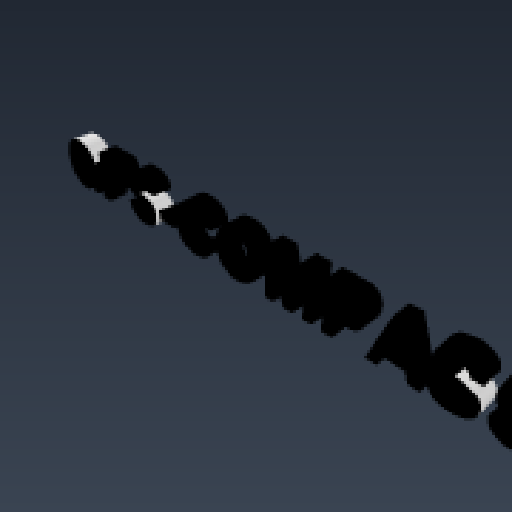
# Autodesk Inventor part: GPS-Compass_name
Saved by Autodesk Inventor 2026.2 (Build 302298000, 298)
## iProperties
Created: 2025-11-27
Part Number: GPS-Compass_name
Material: Generic
Document SubType Name: Modeling
Designer: MenMe
Density: 1 g/cm^3
Appearance: Default
Author: MenMe
Autodesk Inventor part; units mm, degrees
ref_plane "YZ Plane" through (0, 0, 0) normal (1, 0, 0) x (0, 1, 0)
ref_plane "XZ Plane" through (0, 0, 0) normal (0, 1, 0) x (-1, 0, 0)
ref_plane "XY Plane" through (0, 0, 0) normal (0, 0, 1) x (1, 0, 0)
sketch "Sketch2" plane through (0, 0, 0) normal (0, 0, 1) x (1, 0, 0)
  line L0 (0, 0) -> (50, 0) construction
  line L1 (50, 0) -> (50, -7) construction
  line L2 (50, -7) -> (0, -7) construction
  line L3 (0, -7) -> (0, 0) construction
  spline S0 degree 2 poles (4.1164, -4.544) (3.8396, -4.9226) (3.127, -5.2769) (2.6507, -5.2769) knots 0 0 0 1 2 2 2
  spline S1 degree 2 poles (2.6507, -5.2769) (1.6002, -5.2769) (0.2972, -3.8192) (0.2972, -2.6344) knots 0 0 0 1 2 2 2
  spline S2 degree 2 poles (0.2972, -2.6344) (0.2972, -1.4414) (1.5961, -0.0081) (2.6751, -0.0081) knots 0 0 0 1 2 2 2
  spline S3 degree 2 poles (2.6751, -0.0081) (3.6156, -0.0081) (4.8046, -0.908) (4.9186, -1.6938) knots 0 0 0 1 2 2 2
  line L4 (4.9186, -1.6938) -> (3.8681, -1.6938)
  spline S4 degree 2 poles (3.8681, -1.6938) (3.7744, -1.307) (3.184, -0.8998) (2.7117, -0.8998) knots 0 0 0 1 2 2 2
  spline S5 degree 2 poles (2.7117, -0.8998) (2.0847, -0.8998) (1.3681, -1.82) (1.3681, -2.6303) knots 0 0 0 1 2 2 2
  spline S6 degree 2 poles (1.3681, -2.6303) (1.3681, -3.4446) (2.1173, -4.3648) (2.7687, -4.3648) knots 0 0 0 1 2 2 2
  spline S7 degree 2 poles (2.7687, -4.3648) (3.2573, -4.3648) (3.9169, -3.7866) (3.9943, -3.2858) knots 0 0 0 1 2 2 2
  line L5 (3.9943, -3.2858) -> (2.8583, -3.2858)
  line L6 (2.8583, -3.2858) -> (2.8583, -2.4308)
  line L7 (2.8583, -2.4308) -> (4.9308, -2.4308)
  line L8 (4.9308, -2.4308) -> (4.9308, -5.1384)
  line L9 (4.9308, -5.1384) -> (4.2427, -5.1384)
  line L10 (4.2427, -5.1384) -> (4.1164, -4.544)
  line L11 (6.9503, -3.3591) -> (6.9503, -5.1384)
  line L12 (6.9503, -5.1384) -> (5.9202, -5.1384)
  line L13 (5.9202, -5.1384) -> (5.9202, -0.1384)
  line L14 (5.9202, -0.1384) -> (8.1433, -0.1384)
  spline S8 degree 2 poles (8.1433, -0.1384) (8.9332, -0.1384) (9.7435, -0.9568) (9.7435, -1.7467) knots 0 0 0 1 2 2 2
  spline S9 degree 2 poles (9.7435, -1.7467) (9.7435, -2.5204) (8.9495, -3.3591) (8.2125, -3.3591) knots 0 0 0 1 2 2 2
  line L15 (8.2125, -3.3591) -> (6.9503, -3.3591)
  line L16 (6.9585, -2.4511) -> (7.952, -2.4511)
  spline S10 degree 2 poles (7.952, -2.4511) (8.355, -2.4511) (8.7215, -2.1091) (8.7215, -1.7305) knots 0 0 0 1 2 2 2
  spline S11 degree 2 poles (8.7215, -1.7305) (8.7215, -1.3762) (8.3632, -1.0098) (8.0049, -1.0098) knots 0 0 0 1 2 2 2
  line L17 (8.0049, -1.0098) -> (6.9585, -1.0098)
  line L18 (6.9585, -1.0098) -> (6.9585, -2.4511)
  line L19 (10.3298, -3.5912) -> (11.3436, -3.5912)
  spline S12 degree 2 poles (11.3436, -3.5912) (11.4007, -4.0024) (11.9585, -4.4015) (12.4837, -4.4015) knots 0 0 0 1 2 2 2
  spline S13 degree 2 poles (12.4837, -4.4015) (12.9316, -4.4015) (13.3876, -4.0839) (13.3876, -3.7704) knots 0 0 0 1 2 2 2
  spline S14 degree 2 poles (13.3876, -3.7704) (13.3876, -3.3143) (12.0806, -3.013) knots 0 0 0 1 1 1
  spline S15 degree 2 poles (12.0806, -3.013) (12.0603, -3.013) (12.048, -3.009) knots 0 0 0 1 1 1
  spline S16 degree 2 poles (12.048, -3.009) (12.0155, -3.0008) (11.9422, -2.9845) knots 0 0 0 1 1 1
  spline S17 degree 2 poles (11.9422, -2.9845) (11.2459, -2.8298) (10.9446, -2.6425) knots 0 0 0 1 1 1
  spline S18 degree 2 poles (10.9446, -2.6425) (10.68, -2.4715) (10.4031, -1.8974) (10.4031, -1.5065) knots 0 0 0 1 2 2 2
  spline S19 degree 2 poles (10.4031, -1.5065) (10.4031, -0.7777) (11.3925, 0) (12.3331, 0) knots 0 0 0 1 2 2 2
  spline S20 degree 2 poles (12.3331, 0) (13.2085, 0) (14.1938, -0.8306) (14.2223, -1.5839) knots 0 0 0 1 2 2 2
  line L20 (14.2223, -1.5839) -> (13.2329, -1.5839)
  spline S21 degree 2 poles (13.2329, -1.5839) (13.2044, -1.2215) (12.7036, -0.8388) (12.2394, -0.8388) knots 0 0 0 1 2 2 2
  spline S22 degree 2 poles (12.2394, -0.8388) (11.8363, -0.8388) (11.3966, -1.1564) (11.3966, -1.4454) knots 0 0 0 1 2 2 2
  spline S23 degree 2 poles (11.3966, -1.4454) (11.3966, -1.8445) (12.2476, -2.0399) knots 0 0 0 1 1 1
  spline S24 degree 2 poles (12.2476, -2.0399) (12.4796, -2.0969) (12.6099, -2.1254) knots 0 0 0 1 1 1
  spline S25 degree 2 poles (12.6099, -2.1254) (13.1555, -2.2638) (13.6156, -2.4226) (13.7866, -2.5163) knots 0 0 0 1 2 2 2
  spline S26 degree 2 poles (13.7866, -2.5163) (14.092, -2.6873) (14.3974, -3.2451) (14.3974, -3.636) knots 0 0 0 1 2 2 2
  spline S27 degree 2 poles (14.3974, -3.636) (14.3974, -4.4178) (13.3469, -5.2769) (12.386, -5.2769) knots 0 0 0 1 2 2 2
  spline S28 degree 2 poles (12.386, -5.2769) (11.4454, -5.2769) (10.3705, -4.4015) (10.3298, -3.5912) knots 0 0 0 1 2 2 2
  line L21 (14.8941, -3.7541) -> (14.8941, -2.8217)
  line L22 (14.8941, -2.8217) -> (16.8037, -2.8217)
  line L23 (16.8037, -2.8217) -> (16.8037, -3.7541)
  line L24 (16.8037, -3.7541) -> (14.8941, -3.7541)
  spline S29 degree 2 poles (21.8811, -3.4202) (21.8241, -4.2712) (20.623, -5.2769) (19.6621, -5.2769) knots 0 0 0 1 2 2 2
  spline S30 degree 2 poles (19.6621, -5.2769) (18.5505, -5.2769) (17.3168, -3.8925) (17.3168, -2.6425) knots 0 0 0 1 2 2 2
  spline S31 degree 2 poles (17.3168, -2.6425) (17.3168, -1.364) (18.5749, -0.0081) (19.7516, -0.0081) knots 0 0 0 1 2 2 2
  spline S32 degree 2 poles (19.7516, -0.0081) (20.7085, -0.0081) (21.82, -0.9446) (21.873, -1.7956) knots 0 0 0 1 2 2 2
  line L25 (21.873, -1.7956) -> (20.8591, -1.7956)
  spline S33 degree 2 poles (20.8591, -1.7956) (20.794, -1.3681) (20.2321, -0.9243) (19.7516, -0.9243) knots 0 0 0 1 2 2 2
  spline S34 degree 2 poles (19.7516, -0.9243) (19.0717, -0.9243) (18.3673, -1.7997) (18.3673, -2.6425) knots 0 0 0 1 2 2 2
  spline S35 degree 2 poles (18.3673, -2.6425) (18.3673, -3.4568) (19.0717, -4.3445) (19.7191, -4.3445) knots 0 0 0 1 2 2 2
  spline S36 degree 2 poles (19.7191, -4.3445) (20.1873, -4.3445) (20.7818, -3.8681) (20.8713, -3.4202) knots 0 0 0 1 2 2 2
  line L26 (20.8713, -3.4202) -> (21.8811, -3.4202)
  spline S37 degree 2 poles (22.4837, -2.6425) (22.4837, -1.4292) (23.8029, -0.0081) (24.9267, -0.0081) knots 0 0 0 1 2 2 2
  spline S38 degree 2 poles (24.9267, -0.0081) (26.0464, -0.0081) (27.3738, -1.4332) (27.3738, -2.6425) knots 0 0 0 1 2 2 2
  spline S39 degree 2 poles (27.3738, -2.6425) (27.3738, -3.8518) (26.0464, -5.2769) (24.9267, -5.2769) knots 0 0 0 1 2 2 2
  spline S40 degree 2 poles (24.9267, -5.2769) (23.8029, -5.2769) (22.4837, -3.8518) (22.4837, -2.6425) knots 0 0 0 1 2 2 2
  spline S41 degree 2 poles (23.5342, -2.6425) (23.5342, -3.4691) (24.2671, -4.3811) (24.9267, -4.3811) knots 0 0 0 1 2 2 2
  spline S42 degree 2 poles (24.9267, -4.3811) (25.5904, -4.3811) (26.3314, -3.4691) (26.3314, -2.6425) knots 0 0 0 1 2 2 2
  spline S43 degree 2 poles (26.3314, -2.6425) (26.3314, -1.816) (25.5904, -0.9039) (24.9267, -0.9039) knots 0 0 0 1 2 2 2
  spline S44 degree 2 poles (24.9267, -0.9039) (24.2671, -0.9039) (23.5342, -1.8119) (23.5342, -2.6425) knots 0 0 0 1 2 2 2
  line L27 (28.1922, -5.1384) -> (28.1922, -0.1384)
  line L28 (28.1922, -0.1384) -> (29.715, -0.1384)
  line L29 (29.715, -0.1384) -> (30.7125, -3.9454)
  line L30 (30.7125, -3.9454) -> (31.6938, -0.1384)
  line L31 (31.6938, -0.1384) -> (33.2207, -0.1384)
  line L32 (33.2207, -0.1384) -> (33.2207, -5.1384)
  line L33 (33.2207, -5.1384) -> (32.2557, -5.1384)
  line L34 (32.2557, -5.1384) -> (32.2557, -1.1075)
  line L35 (32.2557, -1.1075) -> (31.2419, -5.1384)
  line L36 (31.2419, -5.1384) -> (30.1873, -5.1384)
  line L37 (30.1873, -5.1384) -> (29.1572, -1.1075)
  line L38 (29.1572, -1.1075) -> (29.1572, -5.1384)
  line L39 (29.1572, -5.1384) -> (28.1922, -5.1384)
  line L40 (35.2891, -3.3591) -> (35.2891, -5.1384)
  line L41 (35.2891, -5.1384) -> (34.259, -5.1384)
  line L42 (34.259, -5.1384) -> (34.259, -0.1384)
  line L43 (34.259, -0.1384) -> (36.4821, -0.1384)
  spline S45 degree 2 poles (36.4821, -0.1384) (37.272, -0.1384) (38.0822, -0.9568) (38.0822, -1.7467) knots 0 0 0 1 2 2 2
  spline S46 degree 2 poles (38.0822, -1.7467) (38.0822, -2.5204) (37.2883, -3.3591) (36.5513, -3.3591) knots 0 0 0 1 2 2 2
  line L44 (36.5513, -3.3591) -> (35.2891, -3.3591)
  line L45 (35.2972, -2.4511) -> (36.2907, -2.4511)
  spline S47 degree 2 poles (36.2907, -2.4511) (36.6938, -2.4511) (37.0603, -2.1091) (37.0603, -1.7305) knots 0 0 0 1 2 2 2
  spline S48 degree 2 poles (37.0603, -1.7305) (37.0603, -1.3762) (36.702, -1.0098) (36.3436, -1.0098) knots 0 0 0 1 2 2 2
  line L46 (36.3436, -1.0098) -> (35.2972, -1.0098)
  line L47 (35.2972, -1.0098) -> (35.2972, -2.4511)
  line L48 (40.1629, -0.1384) -> (41.3518, -0.1384)
  line L49 (41.3518, -0.1384) -> (43.1555, -5.1384)
  line L50 (43.1555, -5.1384) -> (42.0765, -5.1384)
  line L51 (42.0765, -5.1384) -> (41.7345, -4.1083)
  line L52 (41.7345, -4.1083) -> (39.7964, -4.1083)
  line L53 (39.7964, -4.1083) -> (39.4666, -5.1384)
  line L54 (39.4666, -5.1384) -> (38.3836, -5.1384)
  line L55 (38.3836, -5.1384) -> (40.1629, -0.1384)
  line L56 (40.7614, -1.1401) -> (40.0692, -3.2655)
  line L57 (40.0692, -3.2655) -> (41.4577, -3.2655)
  line L58 (41.4577, -3.2655) -> (40.7614, -1.1401)
  line L59 (43.4406, -3.5912) -> (44.4544, -3.5912)
  spline S49 degree 2 poles (44.4544, -3.5912) (44.5114, -4.0024) (45.0692, -4.4015) (45.5945, -4.4015) knots 0 0 0 1 2 2 2
  spline S50 degree 2 poles (45.5945, -4.4015) (46.0423, -4.4015) (46.4984, -4.0839) (46.4984, -3.7704) knots 0 0 0 1 2 2 2
  spline S51 degree 2 poles (46.4984, -3.7704) (46.4984, -3.3143) (45.1914, -3.013) knots 0 0 0 1 1 1
  spline S52 degree 2 poles (45.1914, -3.013) (45.171, -3.013) (45.1588, -3.009) knots 0 0 0 1 1 1
  spline S53 degree 2 poles (45.1588, -3.009) (45.1262, -3.0008) (45.0529, -2.9845) knots 0 0 0 1 1 1
  spline S54 degree 2 poles (45.0529, -2.9845) (44.3567, -2.8298) (44.0554, -2.6425) knots 0 0 0 1 1 1
  spline S55 degree 2 poles (44.0554, -2.6425) (43.7907, -2.4715) (43.5138, -1.8974) (43.5138, -1.5065) knots 0 0 0 1 2 2 2
  spline S56 degree 2 poles (43.5138, -1.5065) (43.5138, -0.7777) (44.5033, 0) (45.4438, 0) knots 0 0 0 1 2 2 2
  spline S57 degree 2 poles (45.4438, 0) (46.3192, 0) (47.3046, -0.8306) (47.3331, -1.5839) knots 0 0 0 1 2 2 2
  line L60 (47.3331, -1.5839) -> (46.3436, -1.5839)
  spline S58 degree 2 poles (46.3436, -1.5839) (46.3151, -1.2215) (45.8143, -0.8388) (45.3502, -0.8388) knots 0 0 0 1 2 2 2
  spline S59 degree 2 poles (45.3502, -0.8388) (44.9471, -0.8388) (44.5073, -1.1564) (44.5073, -1.4454) knots 0 0 0 1 2 2 2
  spline S60 degree 2 poles (44.5073, -1.4454) (44.5073, -1.8445) (45.3583, -2.0399) knots 0 0 0 1 1 1
  spline S61 degree 2 poles (45.3583, -2.0399) (45.5904, -2.0969) (45.7207, -2.1254) knots 0 0 0 1 1 1
  spline S62 degree 2 poles (45.7207, -2.1254) (46.2663, -2.2638) (46.7264, -2.4226) (46.8974, -2.5163) knots 0 0 0 1 2 2 2
  spline S63 degree 2 poles (46.8974, -2.5163) (47.2028, -2.6873) (47.5081, -3.2451) (47.5081, -3.636) knots 0 0 0 1 2 2 2
  spline S64 degree 2 poles (47.5081, -3.636) (47.5081, -4.4178) (46.4577, -5.2769) (45.4967, -5.2769) knots 0 0 0 1 2 2 2
  spline S65 degree 2 poles (45.4967, -5.2769) (44.5562, -5.2769) (43.4813, -4.4015) (43.4406, -3.5912) knots 0 0 0 1 2 2 2
  line L61 (48.0822, -3.5912) -> (49.0961, -3.5912)
  spline S66 degree 2 poles (49.0961, -3.5912) (49.1531, -4.0024) (49.7109, -4.4015) (50.2362, -4.4015) knots 0 0 0 1 2 2 2
  spline S67 degree 2 poles (50.2362, -4.4015) (50.684, -4.4015) (51.1401, -4.0839) (51.1401, -3.7704) knots 0 0 0 1 2 2 2
  spline S68 degree 2 poles (51.1401, -3.7704) (51.1401, -3.3143) (49.8331, -3.013) knots 0 0 0 1 1 1
  spline S69 degree 2 poles (49.8331, -3.013) (49.8127, -3.013) (49.8005, -3.009) knots 0 0 0 1 1 1
  spline S70 degree 2 poles (49.8005, -3.009) (49.7679, -3.0008) (49.6946, -2.9845) knots 0 0 0 1 1 1
  spline S71 degree 2 poles (49.6946, -2.9845) (48.9984, -2.8298) (48.6971, -2.6425) knots 0 0 0 1 1 1
  spline S72 degree 2 poles (48.6971, -2.6425) (48.4324, -2.4715) (48.1555, -1.8974) (48.1555, -1.5065) knots 0 0 0 1 2 2 2
  spline S73 degree 2 poles (48.1555, -1.5065) (48.1555, -0.7777) (49.145, 0) (50.0855, 0) knots 0 0 0 1 2 2 2
  spline S74 degree 2 poles (50.0855, 0) (50.9609, 0) (51.9463, -0.8306) (51.9748, -1.5839) knots 0 0 0 1 2 2 2
  line L62 (51.9748, -1.5839) -> (50.9853, -1.5839)
  spline S75 degree 2 poles (50.9853, -1.5839) (50.9568, -1.2215) (50.456, -0.8388) (49.9919, -0.8388) knots 0 0 0 1 2 2 2
  spline S76 degree 2 poles (49.9919, -0.8388) (49.5888, -0.8388) (49.149, -1.1564) (49.149, -1.4454) knots 0 0 0 1 2 2 2
  spline S77 degree 2 poles (49.149, -1.4454) (49.149, -1.8445) (50, -2.0399) knots 0 0 0 1 1 1
  spline S78 degree 2 poles (50, -2.0399) (50.2321, -2.0969) (50.3624, -2.1254) knots 0 0 0 1 1 1
  spline S79 degree 2 poles (50.3624, -2.1254) (50.908, -2.2638) (51.3681, -2.4226) (51.5391, -2.5163) knots 0 0 0 1 2 2 2
  spline S80 degree 2 poles (51.5391, -2.5163) (51.8445, -2.6873) (52.1498, -3.2451) (52.1498, -3.636) knots 0 0 0 1 2 2 2
  spline S81 degree 2 poles (52.1498, -3.636) (52.1498, -4.4178) (51.0993, -5.2769) (50.1384, -5.2769) knots 0 0 0 1 2 2 2
  spline S82 degree 2 poles (50.1384, -5.2769) (49.1979, -5.2769) (48.123, -4.4015) (48.0822, -3.5912) knots 0 0 0 1 2 2 2
  dimension "d0" = 50
  dimension "d1" = 7
  constraints: 1 coincident, 1 horizontal alignment, 2 other
  measures "d0" distance of L0.start L0.end
  measures "d1" distance of L2.end L0.start
extrude "Extrusion1" add sketch "Sketch2" along normal blind 2
body "Solid1"
